Autodesk Fusion 360 part; units mm, degrees
(part 2 of 2)
  spline S157 degree 3 poles (-2.1558, 10.4523) (-2.135, 10.4434) (-2.0932, 10.4255) (-2.0478, 10.423) (-2.025, 10.4217) knots 0 0 0 0 0.006752 0.013527 0.013527 0.013527 0.013527
  spline S158 degree 3 poles (-2.025, 10.4217) (-2.005, 10.4227) (-1.9647, 10.4247) (-1.9267, 10.4381) (-1.9075, 10.4449) knots 0 0 0 0 0.005973 0.012029 0.012029 0.012029 0.012029
  spline S159 degree 3 poles (-1.9075, 10.4449) (-1.8903, 10.4521) (-1.8594, 10.4651) (-1.8325, 10.4853) (-1.8206, 10.4943) knots 0 0 0 0 0.005577 0.010031 0.010031 0.010031 0.010031
  line L54 (-1.8206, 10.4943) -> (-1.8206, 10.6246)
  line L55 (-1.8206, 10.6246) -> (-2.0264, 10.6246)
  line L56 (1.7315, 10.3501) -> (1.7315, 11.0501)
  line L57 (1.7315, 11.0501) -> (1.8241, 11.0501)
  line L58 (1.8241, 11.0501) -> (1.8241, 10.4327)
  line L59 (1.8241, 10.4327) -> (2.1689, 10.4327)
  line L60 (2.1689, 10.4327) -> (2.1689, 10.3501)
  line L61 (2.1689, 10.3501) -> (1.7315, 10.3501)
  line L62 (3.4567, 10.3501) -> (3.4567, 11.0501)
  line L63 (3.4567, 11.0501) -> (3.6979, 11.0501)
  spline S160 degree 3 poles (3.6979, 11.0501) (3.7219, 11.05) (3.7638, 11.0498) (3.805, 11.043) (3.8225, 11.0401) knots 0 0 0 0 0.007203 0.01252 0.01252 0.01252 0.01252
  spline S161 degree 3 poles (3.8225, 11.0401) (3.8416, 11.0347) (3.8789, 11.0242) (3.91, 11.0011) (3.9252, 10.9899) knots 0 0 0 0 0.005905 0.01151 0.01151 0.01151 0.01151
  spline S162 degree 3 poles (3.9252, 10.9899) (3.9425, 10.973) (3.978, 10.9386) (3.9979, 10.8933) (4.008, 10.8703) knots 0 0 0 0 0.0072 0.014672 0.014672 0.014672 0.014672
  spline S163 degree 3 poles (4.008, 10.8703) (4.016, 10.8445) (4.0328, 10.7903) (4.0345, 10.7336) (4.0355, 10.7039) knots 0 0 0 0 0.008068 0.016934 0.016934 0.016934 0.016934
  spline S164 degree 3 poles (4.0355, 10.7039) (4.0349, 10.6787) (4.0337, 10.6309) (4.0223, 10.5845) (4.0168, 10.5626) knots 0 0 0 0 0.007535 0.014294 0.014294 0.014294 0.014294
  spline S165 degree 3 poles (4.0168, 10.5626) (4.0106, 10.5434) (3.9987, 10.5075) (3.9785, 10.4755) (3.9691, 10.4606) knots 0 0 0 0 0.006016 0.011295 0.011295 0.011295 0.011295
  spline S166 degree 3 poles (3.9691, 10.4606) (3.9594, 10.4481) (3.941, 10.4241) (3.9169, 10.4058) (3.9053, 10.3971) knots 0 0 0 0 0.004722 0.009034 0.009034 0.009034 0.009034
  spline S167 degree 3 poles (3.9053, 10.3971) (3.8928, 10.3898) (3.8666, 10.3744) (3.8372, 10.3663) (3.8218, 10.362) knots 0 0 0 0 0.004328 0.009098 0.009098 0.009098 0.009098
  spline S168 degree 3 poles (3.8218, 10.362) (3.8043, 10.3585) (3.7672, 10.3512) (3.7294, 10.3505) (3.7093, 10.3501) knots 0 0 0 0 0.005334 0.011328 0.011328 0.011328 0.011328
  line L64 (3.7093, 10.3501) -> (3.4567, 10.3501)
  line L65 (-6.65, -11.9) -> (6.65, -11.9)
  line L66 (6.65, -11.9) -> (6.65, -13.4)
  line L67 (6.65, -13.4) -> (-6.65, -13.4)
  line L68 (-6.65, -13.4) -> (-6.65, -11.9)
  dimension "d62" = 7.5
  dimension "d63" = 7.5
  dimension "d64" = 1.5
  constraint horizontal L65
  constraint vertical L66
  constraint horizontal L67
  constraint vertical L68
  constraint coincident L12 L66.end
  measures "d62" distance of L9 L66
  measures "d63" distance of L11 L68
  measures "d64" distance of L65 L67
extrude "Extrude7" cut sketch "Sketch6" against normal through all contours L12 L65 L66 L67 L68 bodies 3 in component "Base PCB"
fillet "Fillet2" radius 1.5 2 edges at (-6.65, -11.9, -0.8) (6.65, -11.9, -0.8) on bodies 3 in component "Base PCB"
ref_plane "WorkPlane1" through (0, 0, 0.8) normal (-1, 0, 0) x (0, -1, 0) in component "Base PCB"
sketch "Sketch7" plane through (0, 0, 0.8) normal (-1, 0, 0) x (0, 0, -1) in component "Base PCB"
  line L0 (0.8, 9.6) -> (-0.7, 9.6)
  line L1 (0.05, 9.6) -> (0.05, 12.076)
  spline S0 degree 5 poles (0.05, 12.076) (0.045, 12.144) (0.0386, 12.2766) (0.0397, 12.4652) (0.0626, 12.6958) (0.1271, 12.9492) (0.2274, 13.1673) (0.362, 13.3502) (0.5282, 13.4987) (0.7209, 13.6148) (0.9327, 13.7017) (1.1549, 13.763) (1.3785, 13.8024) (1.5952, 13.823) (1.7983, 13.827) (1.9839, 13.8145) (2.1498, 13.7849) (2.2954, 13.7368) (2.4207, 13.6687) (2.5263, 13.5796) (2.6126, 13.4692) (2.6666, 13.3637) (2.6988, 13.2752) (2.7166, 13.2119) (2.7246, 13.1792) knots 0 0 0 0 0 0 0.05 0.1 0.15 0.2 0.25 0.3 0.35 0.4 0.45 0.5 0.55 0.6 0.65 0.7 0.75 0.8 0.85 0.9 0.95 1 1 1 1 1 1
  line L2 (-0.15, 9.6) -> (-0.15, 12.0687)
  spline S1 degree 3 poles (-0.15, 12.0687) (-0.2001, 12.7431) (-0.0311, 13.2794) (0.344, 13.5973) (0.756, 13.9465) (1.3238, 14.03) (1.7637, 14.0263) (2.2232, 14.0224) (2.6073, 13.8705) (2.81, 13.5324) (2.8632, 13.4437) (2.9043, 13.3456) (2.935, 13.2395) (2.9376, 13.2305) (2.9402, 13.2214) (2.9429, 13.2124) knots 0.001049 0.001049 0.001049 0.001049 0.282713 0.282713 0.282713 0.592043 0.592043 0.592043 0.915235 0.915235 0.915235 1 1 1 1.008325 1.008325 1.008325 1.008325
  line L3 (2.9429, 13.2124) -> (2.9006, 7.1)
  line L4 (2.9006, 7.1) -> (2.7447, 7.1)
  line L5 (2.4, -13.25) -> (2.4, 12.4) construction
  line L6 (2.7447, 7.1) -> (2.4, 7.1) construction
  spline S2 degree 5 poles (2.6, 7.1) (2.6001, 7.112) (2.6003, 7.1388) (2.6012, 7.1874) (2.6028, 7.2697) (2.604, 7.4064) (2.603, 7.581) (2.5995, 7.7938) (2.5954, 8.0386) (2.5945, 8.3035) (2.6011, 8.5745) (2.6192, 8.8383) (2.651, 9.0847) (2.6965, 9.3102) (2.7519, 9.5198) (2.8118, 9.723) (2.8589, 9.8891) (2.8915, 10.0198) (2.9119, 10.1102) (2.9217, 10.1562) knots 0 0 0 0 0 0 0.066667 0.133333 0.2 0.266667 0.333333 0.4 0.466667 0.533333 0.6 0.666667 0.733333 0.8 0.866667 0.933333 1 1 1 1 1 1
  line L7 (2.5992, 6.9502) -> (2.6008, 7.2498)
  line L8 (2.8515, 9.8275) -> (2.992, 10.4849)
  spline S3 degree 3 poles (2.4, 7.1011) (2.4007, 7.2228) (2.4028, 7.4903) (2.3971, 7.9612) (2.3916, 8.4113) (2.4129, 8.965) (2.5099, 9.3762) (2.5794, 9.6707) (2.6648, 9.9108) (2.7262, 10.198) knots 0 0 0 0 0.378704 0.378704 0.378704 0.740683 0.740683 0.740683 1 1 1 1
  line L9 (2.6, 7.1) -> (2.4, 7.1)
  line L10 (2.7246, 13.1792) -> (2.7246, 10.2352)
  line L11 (2.727, 9.4208) -> (2.7447, 7.1)
  line L12 (2.7246, 10.1907) -> (2.727, 9.4208) construction
  spline S4 degree 5 poles (2.7261, 10.198) (2.7261, 10.1995) (2.726, 10.2024) (2.7258, 10.2069) (2.7255, 10.2129) (2.7252, 10.2203) (2.725, 10.2263) (2.7248, 10.2307) (2.7247, 10.2337) (2.7246, 10.2352) knots 0 0 0 0 0 0 0.2 0.4 0.6 0.8 1 1 1 1 1 1
  line L13 (2.7246, 10.2352) -> (2.7246, 10.1907) construction
  line L14 (2.4, 7.1) -> (2.4, 7.1011)
  point P0 (0.4788, 13.4465)
  point P1 (1.5827, 13.8183)
  point P2 (2.3729, 13.6905)
  point P3 (2.4, 13.4)
  point P4 (2.6017, 7.6467)
  point P5 (2.6467, 9.03)
  dimension "d68" = 6.3
  dimension "d70" = 0.2
  dimension "d71" = -0.2
  constraint midpoint L0 L1.start
  constraint perpendicular L0 L1
  constraint vertical L10
  constraint perpendicular L4 L10
  constraint coincident L5 L6.end
  constraint perpendicular L6 L10
  constraint coincident L6 S2.start
  constraint midpoint L3 S2.end
  constraint midpoint S2.start L7
  constraint midpoint S2.end L8
  constraint coincident S3 L12.start
  constraint coincident S2 L11.start
  constraint parallel L1 L2
  constraint vertical L13
  constraint coincident L5 S3.start
  constraint perpendicular L9 L14
  measures "d68" vertical distance of L4.end P3
  measures "d70" distance of L6.end S2.start
extrude "Extrude1'''" add sketch "Sketch7" along normal mid plane 21.75 separate body contours L0 L1 S0 L2 S1 L3 S2 S3 L9 L10 S4 L14 makes body 8 in component "fLEX"
sketch "Sketch1 (4)" plane through (0, 0, 0.95) normal (0, 0, 1) x (1, 0, 0) in component "fLEX"
  line L0 (10.875, -9.6) -> (-10.875, -9.6) construction
  line L1 (-10.875, -9.6) -> (-10.875, -12.0687)
  line L2 (-10.875, -12.0687) -> (10.875, -12.0687)
  line L3 (10.875, -12.0687) -> (10.875, -9.6)
  line L4 (6, -14.0264) -> (-6, -14.0264)
  line L5 (-6, -14.0264) -> (-6, -5.1736)
  line L6 (-6, -5.1736) -> (6, -5.1736)
  line L7 (6, -5.1736) -> (6, -14.0264)
  line L8 (6, -14.0264) -> (-6, -5.1736) construction
  line L9 (-6, -14.0264) -> (6, -5.1736) construction
  line L10 (10.875, -12.0687) -> (-10.875, -12.0687) construction
  line L11 (-10.875, -14.0264) -> (-10.875, -12.0687) construction
  line L12 (-10.875, -13.2124) -> (10.875, -13.2124) construction
  line L13 (10.875, -12.0687) -> (10.875, -14.0264) construction
  line L14 (-10.875, -14.0264) -> (-12.5306, -14.0264) construction
  line L15 (-13.7995, -3.2805) -> (14.151, -3.2805)
  line L16 (14.151, -3.2805) -> (14.151, -17.2558)
  line L17 (14.151, -17.2558) -> (-13.7995, -17.2558)
  line L18 (-13.7995, -17.2558) -> (-13.7995, -3.2805)
  point P0 (0, -9.6)
  dimension "d78" = 12
  constraint horizontal L4
  constraint perpendicular L4 L5
  constraint parallel L4 L6
  constraint parallel L5 L7
  constraint coincident L8 P0
  constraint coincident L9 P0
  constraint midpoint L0 P0
  constraint coincident L11.start L14.start
  constraint perpendicular L11 L14
  constraint collinear L4 L14
  constraint horizontal L15
  constraint vertical L16
  constraint horizontal L17
  constraint vertical L18
  measures "d78" distance of L5.end L6.end
extrude "Extrude2'''" cut sketch "Sketch1 (4)" along normal mid plane 5 bodies 8 in component "fLEX"
sketch "Sketch2 (4)" plane through (0, 0, -1.9246) normal (0, 0, 1) x (1, 0, 0) in component "fLEX"
  line L0 (0, -10.2352) -> (-10.875, -10.2352) construction
  line L1 (-10.875, -10.2352) -> (-10.875, -13.1792) construction
  line L2 (-10.875, -13.1792) -> (10.875, -13.1792) construction
  line L3 (10.875, -13.1792) -> (10.875, -10.2352) construction
  line L4 (10.875, -10.2352) -> (0, -10.2352) construction
  line L5 (-6, -10.8343) -> (-11.75, -10.8343)
  line L6 (-11.75, -10.8343) -> (-11.75, -14.5721)
  line L7 (-11.75, -14.5721) -> (-6, -14.5721)
  line L8 (-6, -14.5721) -> (-6, -10.8343)
  line L9 (-6, -9.6) -> (-6, -12.0687)
  line L10 (6, -10.8343) -> (12.1834, -10.8343)
  line L11 (12.1834, -10.8343) -> (12.1834, -14.8779)
  line L12 (12.1834, -14.8779) -> (6, -14.8779)
  line L13 (6, -14.8779) -> (6, -10.8343)
  line L14 (6, -12.0687) -> (6, -9.6)
  constraint horizontal L5
  constraint vertical L6
  constraint horizontal L7
  constraint vertical L8
  constraint midpoint L5.start L9
  constraint horizontal L10
  constraint vertical L11
  constraint horizontal L12
  constraint vertical L13
  constraint midpoint L10.start L14
extrude "Extrude3'" cut sketch "Sketch2 (4)" along normal blind 3 bodies 8 in component "fLEX"
sketch "Sketch3 (2)" plane through (0, 0.0142, -2.0515) normal (0, 0.006908, -0.999976) x (-1, 0, 0) in component "fLEX"
  line L0 (-10.875, -13.2269) -> (10.875, -13.2269) construction
  line L1 (10.875, -13.2269) -> (10.875, -10.1706) construction
  line L2 (10.875, -10.1706) -> (-10.875, -10.1706) construction
  line L3 (-10.875, -10.1706) -> (-10.875, -13.2269) construction
  line L4 (10.875, -9.0322) -> (6, -13.6648)
  line L5 (6, -13.6648) -> (9.5651, -15.3944)
  line L6 (9.5651, -15.3944) -> (12.6355, -14.5296)
  line L7 (12.6355, -14.5296) -> (12.0546, -12.4672)
  line L8 (12.0546, -12.4672) -> (10.875, -9.0322)
  line L9 (10.875, -7.1123) -> (10.875, -10.1706)
  line L10 (10.875, -9.0322) -> (8.4375, -9.0322)
  line L11 (8.4375, -9.0322) -> (6.375, -11.3485)
  line L12 (6.375, -11.3485) -> (6, -13.6648)
  point P0 (6, -13.6648)
  constraint coincident P0 L4.end
  constraint perpendicular L6 L7
  constraint coincident L4.start L9
  constraint perpendicular L9 L10
extrude "Extrude4'" cut sketch "Sketch3 (2)" against normal blind 1 bodies 8 in component "fLEX"
fillet "Fillet1''" radius 0.5 3 edges at (-6.375, -11.3348, -2.0272) (-8.4375, -9.0204, -1.7463) (-10.875, -9.0204, -1.7463) on bodies 8 in component "fLEX"
mirror "Mirror1" about plane through (0, 0, 0) normal (1, 0, 0) of "Extrude4'", "Fillet1''" in component "fLEX"
sketch "Sketch4 (2)" plane through (0, 0, -1.9246) normal (0, 0, 1) x (1, 0, 0) in component "fLEX"
  line L0 (7.3547, -10.2352) -> (0, -10.2352)
  line L1 (0, -10.2352) -> (-7.3547, -10.2352)
  line L2 (-6, -13.6519) -> (-6, -13.1792)
  line L3 (-6, -13.1792) -> (6, -13.1792)
  line L4 (6, -13.1792) -> (6, -13.6519)
  line L5 (-6, -13.1792) -> (-8.474, -13.1792) construction
  line L6 (6, -13.1792) -> (8.9689, -13.1792) construction
  line L7 (6, -13.6519) -> (6.3517, -11.4793)
  line L8 (6.4719, -11.2267) -> (7.3547, -10.2352)
  line L9 (-7.3547, -10.2352) -> (-6.4719, -11.2267)
  line L10 (-6.3517, -11.4793) -> (-6, -13.6519)
  ellipse E0 centre (6.8453, -11.5592) end of major axis (6.8453, -11.0592) minor radius 0.5 (6.4719, -11.2267) -> (6.3517, -11.4793) ccw
  ellipse E1 centre (-6.8453, -11.5592) end of major axis (-6.8453, -11.0592) minor radius 0.5 (-6.3517, -11.4793) -> (-6.4719, -11.2267) ccw
  line L11 (-6, -13.1792) -> (-6.3517, -11.4793)
  line L12 (6, -13.1792) -> (6.3517, -11.4793)
  constraint coincident L2.end L3.start
  constraint perpendicular L2 L5
  constraint coincident L3.end L4.start
  constraint perpendicular L4 L6
  constraint coincident L10.start L11.end
  constraint coincident L7.end L12.end
extrude "Extrude5'" cut sketch "Sketch4 (2)" against normal blind 1 contours L4 L7 L12 | L2 L10 L11 bodies 8 in component "fLEX"
sketch "Sketch1 (5)" plane through (0, 0, -1.6) normal (0, 0, -1) x (-1, 0, 0) in component "PADS"
  line L0 (6.65, -13.4) -> (13.15, -13.4)
  arc A0 (13.15, -13.4) -> (14.15, -12.4) centre (13.15, -12.4) ccw
  line L1 (14.15, -12.4) -> (14.15, 13.25)
  arc A1 (14.15, 13.25) -> (13.15, 14.25) centre (13.15, 13.25) ccw
  line L2 (13.15, 14.25) -> (-13.15, 14.25)
  arc A2 (-13.15, 14.25) -> (-14.15, 13.25) centre (-13.15, 13.25) ccw
  line L3 (-14.15, 13.25) -> (-14.15, -12.4)
  arc A3 (-14.15, -12.4) -> (-13.15, -13.4) centre (-13.15, -12.4) ccw
  line L4 (-13.15, -13.4) -> (-6.65, -13.4)
  arc A4 (-5.15, -11.9) -> (-6.65, -13.4) centre (-5.15, -13.4) ccw
  line L5 (-5.15, -11.9) -> (5.15, -11.9)
  arc A5 (6.65, -13.4) -> (5.15, -11.9) centre (5.15, -13.4) ccw
  circle A6 centre (1.27, 12.35) radius 0.5
  circle A7 centre (-1.27, 12.35) radius 0.5
  circle A8 centre (3.81, 12.35) radius 0.5
  circle A9 centre (-3.81, 12.35) radius 0.5
  line L6 (-11.575, 13.35) -> (-10.525, 13.35)
  arc A10 (-10.525, 10.8) -> (-10.525, 13.35) centre (-10.525, 12.075) ccw
  line L7 (-10.525, 10.8) -> (-11.575, 10.8)
  arc A11 (-11.575, 13.35) -> (-11.575, 10.8) centre (-11.575, 12.075) ccw
  line L8 (10.525, -9.95) -> (11.575, -9.95)
  arc A12 (11.575, -12.5) -> (11.575, -9.95) centre (11.575, -11.225) ccw
  line L9 (11.575, -12.5) -> (10.525, -12.5)
  arc A13 (10.525, -9.95) -> (10.525, -12.5) centre (10.525, -11.225) ccw
  arc A14 (11.575, 10.8) -> (11.575, 13.35) centre (11.575, 12.075) ccw
  line L10 (11.575, 10.8) -> (10.525, 10.8)
  arc A15 (10.525, 13.35) -> (10.525, 10.8) centre (10.525, 12.075) ccw
  line L11 (10.525, 13.35) -> (11.575, 13.35)
  line L12 (-10.525, -12.5) -> (-11.575, -12.5)
  arc A16 (-11.575, -9.95) -> (-11.575, -12.5) centre (-11.575, -11.225) ccw
  line L13 (-11.575, -9.95) -> (-10.525, -9.95)
  arc A17 (-10.525, -12.5) -> (-10.525, -9.95) centre (-10.525, -11.225) ccw
  line L14 (-10.5, -3.834) -> (-10.1, -3.834)
  line L15 (-10.1, -3.834) -> (-10.1, -6.834)
  line L16 (-10.1, -6.834) -> (-10.5, -6.834)
  line L17 (-10.5, -6.834) -> (-10.5, -3.834)
  line L18 (13.34, -5.4) -> (-13.34, -5.4) construction
  line L19 (-6, -12.1792) -> (6, -12.1792) construction
  line L20 (0, -5.4) -> (0, -15.3707) construction
  line L21 (-9.7759, -6.834) -> (-9.7759, -3.834)
  line L22 (-9.7759, -3.834) -> (-9.3759, -3.834)
  line L23 (-9.3759, -6.834) -> (-9.7759, -6.834)
  line L24 (-9.3759, -3.834) -> (-9.3759, -6.834)
  line L25 (-9.0517, -6.834) -> (-9.0517, -3.834)
  line L26 (-9.0517, -3.834) -> (-8.6517, -3.834)
  line L27 (-8.6517, -6.834) -> (-9.0517, -6.834)
  line L28 (-8.6517, -3.834) -> (-8.6517, -6.834)
  line L29 (-8.3276, -6.834) -> (-8.3276, -3.834)
  line L30 (-8.3276, -3.834) -> (-7.9276, -3.834)
  line L31 (-7.9276, -6.834) -> (-8.3276, -6.834)
  line L32 (-7.9276, -3.834) -> (-7.9276, -6.834)
  line L33 (-7.6034, -6.834) -> (-7.6034, -3.834)
  line L34 (-7.6034, -3.834) -> (-7.2034, -3.834)
  line L35 (-7.2034, -6.834) -> (-7.6034, -6.834)
  line L36 (-7.2034, -3.834) -> (-7.2034, -6.834)
  line L37 (-6.8793, -6.834) -> (-6.8793, -3.834)
  line L38 (-6.8793, -3.834) -> (-6.4793, -3.834)
  line L39 (-6.4793, -6.834) -> (-6.8793, -6.834)
  line L40 (-6.4793, -3.834) -> (-6.4793, -6.834)
  line L41 (-6.1552, -6.834) -> (-6.1552, -3.834)
  line L42 (-6.1552, -3.834) -> (-5.7552, -3.834)
  line L43 (-5.7552, -6.834) -> (-6.1552, -6.834)
  line L44 (-5.7552, -3.834) -> (-5.7552, -6.834)
  line L45 (-5.431, -6.834) -> (-5.431, -3.834)
  line L46 (-5.431, -3.834) -> (-5.031, -3.834)
  line L47 (-5.031, -6.834) -> (-5.431, -6.834)
  line L48 (-5.031, -3.834) -> (-5.031, -6.834)
  line L49 (-4.7069, -6.834) -> (-4.7069, -3.834)
  line L50 (-4.7069, -3.834) -> (-4.3069, -3.834)
  line L51 (-4.3069, -6.834) -> (-4.7069, -6.834)
  line L52 (-4.3069, -3.834) -> (-4.3069, -6.834)
  line L53 (-3.9828, -6.834) -> (-3.9828, -3.834)
  line L54 (-3.9828, -3.834) -> (-3.5828, -3.834)
  line L55 (-3.5828, -6.834) -> (-3.9828, -6.834)
  line L56 (-3.5828, -3.834) -> (-3.5828, -6.834)
  line L57 (-3.2586, -6.834) -> (-3.2586, -3.834)
  line L58 (-3.2586, -3.834) -> (-2.8586, -3.834)
  line L59 (-2.8586, -6.834) -> (-3.2586, -6.834)
  line L60 (-2.8586, -3.834) -> (-2.8586, -6.834)
  line L61 (-2.5345, -6.834) -> (-2.5345, -3.834)
  line L62 (-2.5345, -3.834) -> (-2.1345, -3.834)
  line L63 (-2.1345, -6.834) -> (-2.5345, -6.834)
  line L64 (-2.1345, -3.834) -> (-2.1345, -6.834)
  line L65 (-1.8103, -6.834) -> (-1.8103, -3.834)
  line L66 (-1.8103, -3.834) -> (-1.4103, -3.834)
  line L67 (-1.4103, -6.834) -> (-1.8103, -6.834)
  line L68 (-1.4103, -3.834) -> (-1.4103, -6.834)
  line L69 (-1.0862, -6.834) -> (-1.0862, -3.834)
  line L70 (-1.0862, -3.834) -> (-0.6862, -3.834)
  line L71 (-0.6862, -6.834) -> (-1.0862, -6.834)
  line L72 (-0.6862, -3.834) -> (-0.6862, -6.834)
  line L73 (-0.3621, -6.834) -> (-0.3621, -3.834)
  line L74 (-0.3621, -3.834) -> (0.0379, -3.834)
  line L75 (0.0379, -6.834) -> (-0.3621, -6.834)
  line L76 (0.0379, -3.834) -> (0.0379, -6.834)
  line L77 (0.3621, -6.834) -> (0.3621, -3.834)
  line L78 (0.3621, -3.834) -> (0.7621, -3.834)
  line L79 (0.7621, -6.834) -> (0.3621, -6.834)
  line L80 (0.7621, -3.834) -> (0.7621, -6.834)
  line L81 (1.0862, -6.834) -> (1.0862, -3.834)
  line L82 (1.0862, -3.834) -> (1.4862, -3.834)
  line L83 (1.4862, -6.834) -> (1.0862, -6.834)
  line L84 (1.4862, -3.834) -> (1.4862, -6.834)
  line L85 (1.8103, -6.834) -> (1.8103, -3.834)
  line L86 (1.8103, -3.834) -> (2.2103, -3.834)
  line L87 (2.2103, -6.834) -> (1.8103, -6.834)
  line L88 (2.2103, -3.834) -> (2.2103, -6.834)
  line L89 (2.5345, -6.834) -> (2.5345, -3.834)
  line L90 (2.5345, -3.834) -> (2.9345, -3.834)
  line L91 (2.9345, -6.834) -> (2.5345, -6.834)
  line L92 (2.9345, -3.834) -> (2.9345, -6.834)
  line L93 (3.2586, -6.834) -> (3.2586, -3.834)
  line L94 (3.2586, -3.834) -> (3.6586, -3.834)
  line L95 (3.6586, -6.834) -> (3.2586, -6.834)
  line L96 (3.6586, -3.834) -> (3.6586, -6.834)
  line L97 (3.9828, -6.834) -> (3.9828, -3.834)
  line L98 (3.9828, -3.834) -> (4.3828, -3.834)
  line L99 (4.3828, -6.834) -> (3.9828, -6.834)
  line L100 (4.3828, -3.834) -> (4.3828, -6.834)
  line L101 (4.7069, -6.834) -> (4.7069, -3.834)
  line L102 (4.7069, -3.834) -> (5.1069, -3.834)
  line L103 (5.1069, -6.834) -> (4.7069, -6.834)
  line L104 (5.1069, -3.834) -> (5.1069, -6.834)
  line L105 (5.431, -6.834) -> (5.431, -3.834)
  line L106 (5.431, -3.834) -> (5.831, -3.834)
  line L107 (5.831, -6.834) -> (5.431, -6.834)
  line L108 (5.831, -3.834) -> (5.831, -6.834)
  line L109 (6.1552, -6.834) -> (6.1552, -3.834)
  line L110 (6.1552, -3.834) -> (6.5552, -3.834)
  line L111 (6.5552, -6.834) -> (6.1552, -6.834)
  line L112 (6.5552, -3.834) -> (6.5552, -6.834)
  line L113 (6.8793, -6.834) -> (6.8793, -3.834)
  line L114 (6.8793, -3.834) -> (7.2793, -3.834)
  line L115 (7.2793, -6.834) -> (6.8793, -6.834)
  line L116 (7.2793, -3.834) -> (7.2793, -6.834)
  line L117 (7.6034, -6.834) -> (7.6034, -3.834)
  line L118 (7.6034, -3.834) -> (8.0034, -3.834)
  line L119 (8.0034, -6.834) -> (7.6034, -6.834)
  line L120 (8.0034, -3.834) -> (8.0034, -6.834)
  line L121 (8.3276, -6.834) -> (8.3276, -3.834)
  line L122 (8.3276, -3.834) -> (8.7276, -3.834)
  line L123 (8.7276, -6.834) -> (8.3276, -6.834)
  line L124 (8.7276, -3.834) -> (8.7276, -6.834)
  line L125 (9.0517, -6.834) -> (9.0517, -3.834)
  line L126 (9.0517, -3.834) -> (9.4517, -3.834)
  line L127 (9.4517, -6.834) -> (9.0517, -6.834)
  line L128 (9.4517, -3.834) -> (9.4517, -6.834)
  line L129 (9.7759, -6.834) -> (9.7759, -3.834)
  line L130 (9.7759, -3.834) -> (10.1759, -3.834)
  line L131 (10.1759, -6.834) -> (9.7759, -6.834)
  line L132 (10.1759, -3.834) -> (10.1759, -6.834)
  line L133 (10.5, -6.834) -> (10.5, -3.834)
  line L134 (10.5, -3.834) -> (10.9, -3.834)
  line L135 (10.9, -6.834) -> (10.5, -6.834)
  line L136 (10.9, -3.834) -> (10.9, -6.834)
  dimension "d98" = 0.4
  dimension "d99" = 3
  dimension "d100" = 10.5
  dimension "d103" = -21
  dimension "d104" = 0
  constraint horizontal L14
  constraint vertical L15
  constraint horizontal L16
  constraint vertical L17
  constraint midpoint L18 L20.start
  constraint perpendicular L19 L20
  measures "d98" distance of L14.start L14.end
  measures "d99" distance of L14.start L16.end
  measures "d100" distance of L17 L20
extrude "Extrude1''''" add sketch "Sketch1 (5)" along normal blind 0.1 separate body contours L14 L15 L16 L17 makes body 9 in component "PADS"
pattern_linear "R-Pattern1'" count 30 spacing 0.7069 along (-1, 0, 0) of bodies 9 makes body 10 at (9.6598, -4.834, -1.6) makes body 11 at (8.9529, -4.834, -1.6) makes body 12 at (8.246, -4.834, -1.6) makes body 13 at (7.5391, -4.834, -1.6) makes body 14 at (6.8322, -4.834, -1.6) makes body 15 at (6.1253, -4.834, -1.6) makes body 16 at (5.4184, -4.834, -1.6) makes body 17 at (4.7115, -4.834, -1.6) makes body 18 at (4.0046, -4.834, -1.6) makes body 19 at (3.2977, -4.834, -1.6) makes body 20 at (2.5908, -4.834, -1.6) makes body 21 at (1.8839, -4.834, -1.6) makes body 22 at (1.177, -4.834, -1.6) makes body 23 at (0.4701, -4.834, -1.6) makes body 24 at (-0.2368, -4.834, -1.6) makes body 25 at (-0.9437, -4.834, -1.6) makes body 26 at (-1.6506, -4.834, -1.6) makes body 27 at (-2.3575, -4.834, -1.6) makes body 28 at (-3.0644, -4.834, -1.6) makes body 29 at (-3.7713, -4.834, -1.6) makes body 30 at (-4.4782, -4.834, -1.6) makes body 31 at (-5.1851, -4.834, -1.6) makes body 32 at (-5.892, -4.834, -1.6) makes body 33 at (-6.5989, -4.834, -1.6) makes body 34 at (-7.3057, -4.834, -1.6) makes body 35 at (-8.0126, -4.834, -1.6) makes body 36 at (-8.7195, -4.834, -1.6) makes body 37 at (-9.4264, -4.834, -1.6) makes body 38 at (-10.1333, -4.834, -1.6) in component "PADS"
sketch "Sketch1 (6)" plane through (0, 0, -1.6) normal (0, 0, -1) x (-1, 0, 0) in component "res"
  line L0 (6.65, -13.4) -> (13.15, -13.4) construction
  arc A0 (13.15, -13.4) -> (14.15, -12.4) centre (13.15, -12.4) ccw construction
  line L1 (14.15, -12.4) -> (14.15, 13.25) construction
  arc A1 (14.15, 13.25) -> (13.15, 14.25) centre (13.15, 13.25) ccw construction
  line L2 (13.15, 14.25) -> (-13.15, 14.25) construction
  arc A2 (-13.15, 14.25) -> (-14.15, 13.25) centre (-13.15, 13.25) ccw construction
  line L3 (-14.15, 13.25) -> (-14.15, -12.4) construction
  arc A3 (-14.15, -12.4) -> (-13.15, -13.4) centre (-13.15, -12.4) ccw construction
  line L4 (-13.15, -13.4) -> (-6.65, -13.4) construction
  arc A4 (-5.15, -11.9) -> (-6.65, -13.4) centre (-5.15, -13.4) ccw construction
  line L5 (-5.15, -11.9) -> (5.15, -11.9) construction
  arc A5 (6.65, -13.4) -> (5.15, -11.9) centre (5.15, -13.4) ccw construction
  circle A6 centre (1.27, 12.35) radius 0.5 construction
  circle A7 centre (-1.27, 12.35) radius 0.5 construction
  circle A8 centre (3.81, 12.35) radius 0.5 construction
  circle A9 centre (-3.81, 12.35) radius 0.5 construction
  line L6 (-11.575, 13.35) -> (-10.525, 13.35) construction
  arc A10 (-10.525, 10.8) -> (-10.525, 13.35) centre (-10.525, 12.075) ccw construction
  line L7 (-10.525, 10.8) -> (-11.575, 10.8) construction
  arc A11 (-11.575, 13.35) -> (-11.575, 10.8) centre (-11.575, 12.075) ccw construction
  line L8 (10.525, -9.95) -> (11.575, -9.95) construction
  arc A12 (11.575, -12.5) -> (11.575, -9.95) centre (11.575, -11.225) ccw construction
  line L9 (11.575, -12.5) -> (10.525, -12.5) construction
  arc A13 (10.525, -9.95) -> (10.525, -12.5) centre (10.525, -11.225) ccw construction
  arc A14 (11.575, 10.8) -> (11.575, 13.35) centre (11.575, 12.075) ccw construction
  line L10 (11.575, 10.8) -> (10.525, 10.8) construction
  arc A15 (10.525, 13.35) -> (10.525, 10.8) centre (10.525, 12.075) ccw construction
  line L11 (10.525, 13.35) -> (11.575, 13.35) construction
  line L12 (-10.525, -12.5) -> (-11.575, -12.5) construction
  arc A16 (-11.575, -9.95) -> (-11.575, -12.5) centre (-11.575, -11.225) ccw construction
  line L13 (-11.575, -9.95) -> (-10.525, -9.95) construction
  arc A17 (-10.525, -12.5) -> (-10.525, -9.95) centre (-10.525, -11.225) ccw construction
  line L14 (0.4, -0.625) -> (-0.4, -0.625)
  line L15 (-0.4, -0.625) -> (-0.4, 0.625)
  line L16 (-0.4, 0.625) -> (0.4, 0.625)
  line L17 (0.4, 0.625) -> (0.4, -0.625)
  line L18 (0.4, -0.625) -> (-0.4, 0.625) construction
  line L19 (-0.4, -0.625) -> (0.4, 0.625) construction
  dimension "d111" = 1.25
  dimension "d112" = 0.8
  constraint horizontal L14
  constraint perpendicular L14 L15
  constraint parallel L14 L16
  constraint parallel L15 L17
  constraint coincident L18 origin
  constraint coincident L19 origin
  measures "d111" distance of L14.end L15.end
  measures "d112" distance of L15.end L16.end
extrude "Extrude1'''''" add sketch "Sketch1 (6)" along normal blind 0.8 separate body makes body 39 in component "res"
sketch "Sketch2 (5)" plane through (0, 0.625, 0) normal (0, 1, 0) x (-1, 0, 0) in component "res"
  line L0 (0.4, -1.6) -> (-0.4, -1.6)
  line L1 (-0.4, -1.6) -> (-0.4, -2.4)
  line L2 (-0.4, -2.4) -> (0.4, -2.4)
  line L3 (0.4, -2.4) -> (0.4, -1.6)
  line L4 (0.41, -2.41) -> (0.41, -1.59)
  line L5 (0.41, -1.59) -> (-0.41, -1.59)
  line L6 (-0.41, -1.59) -> (-0.41, -2.41)
  line L7 (-0.41, -2.41) -> (0.41, -2.41)
  line L8 (1.4523, -2.4) -> (-0.7053, -2.4)
  dimension "d115" = 0.01
  constraint perpendicular L6 L8
  constraint collinear L2 L8
extrude "Extrude2''''" add sketch "Sketch2 (5)" against normal blind 0.25 contours L0 L1 L3 L4 L5 L6 L8 bodies 39 in component "res"
ref_plane "WorkPlane1" through (0, 0, -1.995) normal (0, 1, 0) x (1, 0, 0) in component "res"
mirror "Mirror1'" about plane through (0, 0, -1.995) normal (0, 1, 0) of "Extrude2''''" in component "res"
pattern_linear "48" [suppressed] in component "Resistores SMD"
fillet "Fillet1'''" radius 0.5 4 edges at (-13.34, 9.6, 0.8) (13.34, 9.6, 0.8) (13.34, -9.6, 0.75) (-13.34, -9.6, 0.75) on bodies 2 in component "Pantalla"
sketch "Sketch3 (3)" plane through (0, 0, -2.4) normal (0, 0, -1) x (-1, 0, 0) in component "res"
  line L0 (0.41, 0.625) -> (-0.41, 0.625) construction
  line L1 (-0.41, 0.625) -> (-0.41, 0.375) construction
  line L2 (-0.41, 0.375) -> (-0.4, 0.375) construction
  line L3 (-0.4, 0.375) -> (-0.4, -0.375) construction
  line L4 (-0.4, -0.375) -> (-0.41, -0.375) construction
  line L5 (-0.41, -0.375) -> (-0.41, -0.625) construction
  line L6 (-0.41, -0.625) -> (0.41, -0.625) construction
  line L7 (0.41, -0.625) -> (0.41, -0.375) construction
  line L8 (0.41, -0.375) -> (0.4, -0.375) construction
  line L9 (0.4, -0.375) -> (0.4, 0.375) construction
  line L10 (0.4, 0.375) -> (0.41, 0.375) construction
  line L11 (0.41, 0.375) -> (0.41, 0.625) construction
  line L12 (-0.51, 0.825) -> (0.51, 0.825)
  line L13 (0.51, 0.825) -> (0.51, -0.825)
  line L14 (0.51, -0.825) -> (-0.51, -0.825)
  line L15 (-0.51, -0.825) -> (-0.51, 0.825)
  line L16 (-0.51, 0.825) -> (0.51, -0.825) construction
  line L17 (0.51, 0.825) -> (-0.51, -0.825) construction
  line L18 (0.51, -0.275) -> (-0.51, -0.275)
  line L19 (0, 0) -> (-0.7339, 0) construction
  line L20 (0.51, 0.275) -> (-0.51, 0.275)
  dimension "d134" = 0.1
  dimension "d135" = 0.2
  dimension "d136" = 0.1
  constraint horizontal L12
  constraint perpendicular L12 L13
  constraint parallel L12 L14
  constraint parallel L13 L15
  constraint coincident L16 L19.start
  constraint coincident L17 L19.start
  constraint coincident L19.start origin
  constraint coincident L13 L18.start
  constraint coincident L15 L18.end
  constraint perpendicular L15 L18
  constraint perpendicular L3 L19
  constraint symmetric L18.start L19 L20.start
  constraint symmetric L18.end L19 L20.end
  measures "d134" distance of L7 L13
  measures "d135" distance of L6 L14
  measures "d136" distance of L3.end L18
extrude "Extrude3''" add sketch "Sketch3 (3)" against normal blind 0.1 contours L12 L13 L15 L20 | L13 L14 L15 L18 bodies 39 in component "res"
fillet "Fillet1''''" radius 0.2 tangency weight 0.8 2 edges at (0, 0.625, -2.3) (0, -0.625, -2.3) on bodies 39 in component "res"
fillet "Fillet2'" radius 0.1 7 edges at (-0.51, -0.825, -2.35) (0.51, 0.825, -2.35) (0.51, 0.275, -2.35) (0.51, -0.275, -2.35) (0.51, -0.825, -2.35) (-0.51, 0.275, -2.35) (-0.51, 0.825, -2.35) on bodies 39 in component "res"
component "Pantalla" placed x (1, 0, 0) y (0, 1, 0) z (0, 0, 1) at (0, 0.525, 0)
component "Base PCB" placed x (1, 0, 0) y (0, 1, 0) z (0, 0, 1) at (0, 0, 0)
component "PINOS" placed x (1, 0, 0) y (0, 1, 0) z (0, 0, 1) at (0, 0, 0)
component "fLEX" placed x (1, 0, 0) y (0, 1, 0) z (0, 0, 1) at (0, 1.525, -0.1)
component "Resistores SMD" placed x (1, 0, 0) y (0, 1, 0) z (0, 0, 1) at (0, 0, 0)
component "PADS" placed x (1, 0, 0) y (0, 1, 0) z (0, 0, 1) at (0, 0, 0) in component "Base PCB"
component "res" placed x (1, 0, 0) y (0, -1, 0) z (0, 0, -1) at (13, 2.425, -4) in component "Resistores SMD"
component "res" placed x (1, 0, 0) y (0, -1, 0) z (0, 0, -1) at (10.1111, 2.425, -4) in component "Resistores SMD"
component "res" placed x (1, 0, 0) y (0, -1, 0) z (0, 0, -1) at (7.2222, 2.425, -4) in component "Resistores SMD"
component "res" placed x (1, 0, 0) y (0, -1, 0) z (0, 0, -1) at (4.3333, 2.425, -4) in component "Resistores SMD"
component "res" placed x (1, 0, 0) y (0, -1, 0) z (0, 0, -1) at (1.4444, 2.425, -4) in component "Resistores SMD"
component "res" placed x (1, 0, 0) y (0, -1, 0) z (0, 0, -1) at (-1.4444, 2.425, -4) in component "Resistores SMD"
component "res" placed x (1, 0, 0) y (0, -1, 0) z (0, 0, -1) at (-4.3333, 2.425, -4) in component "Resistores SMD"
component "res" placed x (1, 0, 0) y (0, -1, 0) z (0, 0, -1) at (-7.2222, 2.425, -4) in component "Resistores SMD"
component "res" placed x (1, 0, 0) y (0, -1, 0) z (0, 0, -1) at (-10.1111, 2.425, -4) in component "Resistores SMD"
component "res" placed x (1, 0, 0) y (0, -1, 0) z (0, 0, -1) at (-13, 2.425, -4) in component "Resistores SMD"
component "res" placed x (0, -1, 0) y (-1, 0, 0) z (0, 0, -1) at (0, -1.575, -4) in component "Resistores SMD"
equation "d11 = ( d9 - 26.68 mm ) / 2"
equation "d14 = ( 2.35 / 2 ) * 1 mm"
equation "d15 = 3.4 mm - ( d14 * 2 )"
equation "d25 = ( 2.54 / 2 ) * 1 mm"
equation "d26 = d25 * 2"
equation "d63 = d62"
equation "d72 = ( 21.75 / 2 ) * 1 mm"
